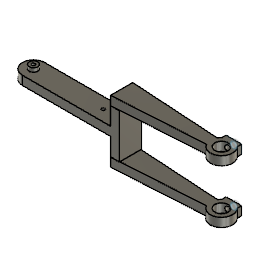
link_2_end_effector (Autodesk Fusion 360 design; units mm, degrees)
Autodesk Fusion 360 part; units mm, degrees
sketch "Sketch1" plane through (0, 0, 0) normal (0, 0, 1) x (1, 0, 0)
  circle A0 centre (-60, 0) radius 3.75 construction
  circle A1 centre (-60, 0) radius 10 construction
  line L0 (-120, 10) -> (-40.6913, 10)
  line L1 (-120, -10) -> (-40.6913, -10)
  line L2 (-40.6913, 10) -> (-40.6913, -10)
  arc A2 (-120, 10) -> (-120, -10) centre (-120, 0) ccw
  dimension "d1" = 20
  dimension "d2" = 7.5
  dimension "d3" = 60
  dimension "d4" = 20
  constraint concentric A0 A1
  constraint tangent L0 A2
  constraint horizontal L0
  constraint tangent L1 A2
  constraint parallel L0 L1
  constraint perpendicular L1 L2
  measures "d1" diameter of A2
  measures "d2" diameter of A0
  measures "d3" distance of A2.centre A0.centre
  measures "d4" diameter of A1
extrude "Extrude1" add sketch "Sketch1" along normal blind 8 makes body 1
sketch "Sketch2" plane through (0, 0, 0) normal (0, 1, 0) x (1, 0, 0)
  line L0 (-43, -20) -> (-35, -20)
  line L1 (-35, -20) -> (-35, 20)
  line L2 (-35, 20) -> (-43, 20)
  line L3 (-43, 20) -> (-43, -20)
  dimension "d7" = 8
  dimension "d8" = 40
  constraint horizontal L0
  constraint vertical L1
  constraint horizontal L2
  constraint vertical L3
  measures "d7" distance of L1 L3
  measures "d8" distance of L0 L2
extrude "Extrude2" add sketch "Sketch2" along normal blind 10 and the other way blind 10 separate body makes body 2
copy_body "Body->Comp1" bodies 1 removing the originals makes body 3 in component "section 1 (l4)"
copy_body "Body->Comp2" bodies 2 removing the originals makes body 4 in component "middle bit"
sketch "Sketch3" plane through (0, 0, 8) normal (0, 0, 1) x (-1, 0, 0)
  line L0 (40.6913, -10) -> (120, -10)
  arc A0 (120, -10) -> (120, 10) centre (120, 0) ccw
  line L1 (120, 10) -> (40.6913, 10)
  line L2 (40.6913, 10) -> (40.6913, -10)
  line L3 (25, -10) -> (25, 10)
  line L4 (25, -10) -> (-56.3022, -4.9345)
  line L5 (25, 10) -> (-56.3022, 4.9345)
  line L6 (-58, -11) -> (-72.0708, -11)
  line L7 (-72.0708, -11) -> (-72.0708, -7.0714)
  line L8 (-58, -7.0714) -> (-58, -11)
  arc A1 (-58, -7.1414) -> (-56.3022, -4.9345) centre (-65, 0) ccw
  arc A2 (-56.3022, 4.9345) -> (-72.0708, -7.0714) centre (-65, 0) ccw
  circle A3 centre (-65, 0) radius 6
  dimension "d17" = 20
  dimension "d18" = 90
  dimension "d19" = 12
  constraint vertical L3
  constraint coincident L5.end A1
  constraint horizontal L6
  constraint vertical L7
  constraint vertical L8
  constraint coincident L8 A1.start
  constraint concentric A1 A2
  constraint concentric A2 A3
  measures "d17" diameter of A1
  measures "d18" distance of A1.centre L3
  measures "d19" diameter of A3
extrude "Extrude3" add sketch "Sketch3" along normal blind 8 separate body contours L3 L4 L5 L6 L7 L8 A1 A2 makes body 5
sketch "Sketch5" plane through (0, 0, 0) normal (0, 0, 1) x (1, 0, 0)
  circle A0 centre (65.005, -0.1371) radius 6
  line L0 (-25, -10) -> (-25, 10)
  line L1 (-25, 10) -> (56.3881, 4.9373)
  line L2 (-25, -10) -> (56.247, -4.9638)
  line L3 (71.9058, 7.1002) -> (72, 7.1002)
  line L4 (72, 7.1002) -> (72, 11)
  line L5 (72, 11) -> (58.1042, 11)
  line L6 (58.1042, 11) -> (58.1042, 7.1002)
  arc A1 (56.247, -4.9638) -> (71.9058, 7.1002) centre (65.005, -0.1371) ccw
  arc A2 (58.1042, 7.1002) -> (56.3881, 4.9373) centre (65.005, -0.1371) ccw
  dimension "d24" = 20
  dimension "d25" = 12
  constraint concentric A0 A1
  constraint vertical L0
  constraint horizontal L3
  constraint vertical L4
  constraint horizontal L5
  constraint vertical L6
  constraint coincident L6.end A1
  constraint concentric A1 A2
  measures "d24" diameter of A1
  measures "d25" diameter of A0
extrude "Extrude4" add sketch "Sketch5" against normal blind 8 separate body makes body 6
copy_body "Body->Comp3" bodies 5 removing the originals makes body 7 in component "top arm "
copy_body "Body->Comp4" bodies 6 removing the originals makes body 8 in component "bottom arm"
cylinder "CylinderPrimitive1" add diameter 7.7 height 3.5 placed x (1, 0, 0) y (0, 1, 0) z (0, 0, 1) at (-120, 0, 8) bodies 3 in component "section 1 (l4)"
cylinder "CylinderPrimitive2" add diameter 7.7 height 3.5 placed x (0, 1, 0) y (1, 0, 0) z (0, 0, -1) at (-57.218, 0, 0) bodies 3 in component "section 1 (l4)"
sketch "Sketch9" plane through (-0.218, 11, 0) normal (0, 1, 0) x (-1, 0, 0)
  line L0 (-54.2887, 20) -> (-40.218, 20)
  line L1 (-40.218, 20) -> (-40.218, 28)
  line L2 (-40.218, 28) -> (-54.2887, 28)
  line L3 (-54.2887, 28) -> (-54.2887, 20)
  circle A0 centre (-47.1099, 23.7364) radius 2.5
  circle A1 centre (-47.2533, -23.9842) radius 2.5
  dimension "d44" = 5
  dimension "d45" = 5
  measures "d44" diameter of A0
  measures "d45" diameter of A1
extrude "Extrude1'" cut sketch "Sketch9" against normal blind 10 contours A0 | A1 sketch seen with x (1, 0, 0) y (0, 1, 0) z (0, 0, 1) at (18, 0, -12) bodies 7 in component "top arm "
extrude "Extrude1''" cut sketch "Sketch9" against normal blind 10 contours A0 | A1 sketch seen with x (1, 0, 0) y (0, 1, 0) z (0, 0, 1) at (18, 0, 20) bodies 8 in component "bottom arm"
combine "Combine1" operation add target body 3 tool bodies 7 8 4 body 7 seen with x (1, 0, 0) y (0, 1, 0) z (0, 0, 1) at (-15.6913, 0, 16) body 8 seen with x (1, 0, 0) y (0, 1, 0) z (0, 0, 1) at (-15.6913, 0, -16) body 4 seen with x (1, 0, 0) y (0, 1, 0) z (0, 0, 1) at (2.3087, 0, 4) in component "section 1 (l4)"
sketch "Sketch10" plane through (0, 0, 7.5) normal (0, 0, 1) x (-1, 0, 0)
  circle A0 centre (122.3087, 0) radius 3.85
  circle A1 centre (122.3087, 0) radius 1.5
  dimension "d50" = 3
  constraint concentric A0 A1
  measures "d50" diameter of A1
extrude "Extrude1'''" cut sketch "Sketch10" against normal blind 18 contours A1 sketch seen with x (1, 0, 0) y (0, 1, 0) z (0, 0, 1) at (2.3087, 0, 4) bodies 3 in component "section 1 (l4)"
sketch "Sketch11" plane through (0, 0, -7.5) normal (0, 0, -1) x (1, 0, 0)
  circle A0 centre (-59.5266, 0) radius 3.85
  circle A1 centre (-59.5266, 0) radius 1.5
  dimension "d53" = 3
  constraint concentric A0 A1
  measures "d53" diameter of A1
extrude "Extrude2'" cut sketch "Sketch11" against normal blind 14 contours A1 sketch seen with x (1, 0, 0) y (0, 1, 0) z (0, 0, 1) at (2.3087, 0, 4) bodies 3 in component "section 1 (l4)"
component "section 1 (l4)" placed x (1, 0, 0) y (0, 1, 0) z (0, 0, 1) at (-2.3087, 0, -4)
component "middle bit" placed x (1, 0, 0) y (0, 1, 0) z (0, 0, 1) at (0, 0, 0)
component "top arm " placed x (1, 0, 0) y (0, 1, 0) z (0, 0, 1) at (-18, 0, 12)
component "bottom arm" placed x (1, 0, 0) y (0, 1, 0) z (0, 0, 1) at (-18, 0, -20)
named bodies: "section 1 (l4)", "middle bit", "top arm", "bottom arm"
